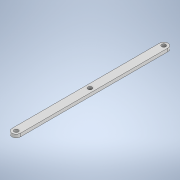
# Autodesk Inventor part: tussenarmen_sturen
Saved by Autodesk Inventor 2022 (Build 260153000, 153)
## iProperties
Created: 2021-12-08
Part Number: tussenarmen_sturen
Material: Generic
Document SubType Name: Modeling
Designer: keemi
Density: 1 g/cm^3
Appearance: Default
Author: keemi
Autodesk Inventor part; units mm, degrees
ref_plane "YZ Plane" through (0, 0, 0) normal (1, 0, 0) x (0, 1, 0)
ref_plane "XZ Plane" through (0, 0, 0) normal (0, 1, 0) x (-1, 0, 0)
ref_plane "XY Plane" through (0, 0, 0) normal (0, 0, 1) x (1, 0, 0)
sketch "Sketch1" plane through (0, 0, 0) normal (0, 1, 0) x (-1, 0, 0)
  circle A0 centre (0, 0) radius 2
  line L0 (0, 0) -> (0, -140)
  circle A1 centre (0, -140) radius 2
  circle A2 centre (0, -140) radius 4
  circle A3 centre (0, 0) radius 4
  line L1 (4, 0) -> (4, -140)
  line L2 (-4, 0) -> (-4, -140)
  line L3 (0, 0) -> (0, -70)
  circle A4 centre (0, -70) radius 2
  dimension "d0" = 4
  dimension "d1" = 140
  dimension "d2" = 4
  dimension "d3" = 8
  dimension "d4" = 8
  dimension "d7" = 70
  dimension "d8" = 4
  constraints: 8 end point, 5 centre point, 5 coincident, 4 point on circle, 2 tangent, 1 midpoint, 1 vertical
  measures "d0" diameter of A0
  measures "d1" distance of L0.start L0.end
  measures "d2" diameter of A1
  measures "d3" diameter of A2
  measures "d4" diameter of A3
  measures "d7" distance of L3.start L3.end
  measures "d8" diameter of A4
extrude "Extrusion1" add sketch "Sketch1" along normal blind 3 contours A3 | A3 L1 A2 L0 A4 | L0 A4 A2 L2 A3 | A2
body "Solid1"
